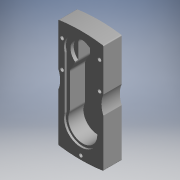
# Autodesk Inventor part: 2610112 EAMM-U-70-D40-...-173---(OT)
Saved by Autodesk Inventor 2017.3 (Build 213256000, 256)
## iProperties
Part Number: 2610112 EAMM-U-70-D40-...-173---(OT)
Material: Generic
Catalog Web Link: www.cadenas.de
Description: EAMM-U---(OT)-Fousing top part
Vendor: FESTO
Document SubType Name: Modeling
Designer: partserver
Manufacturer: FESTO
Mass: 199.697 g
Surface Area: 497.172 cm^2
Volume: 199.697 cm^3
Density: 1 g/cm^3
Appearance: PSOLRGB-192-192-192
Category: PARTsolutions
Company: FESTO
Title: 2610112 EAMM-U-70-D40-...-173---(OT)
Author: Cadenas PARTsolutions
Comments: Fousing top part
PSOL_IDENT_0: {$CADENAS_DATA\23d-libs\festo\parts\e\eamm\parts\eamm_u_ot.prj},220 {VTYP=3D},{NB=2610112 EAMM-U-70-
PSOL_IDENT_1: D40-...-173---(OT)},{LINA=2610112 EAMM-U-70-D40-...-173---(OT)},{NN=EAMM-U---(OT)},{DATE=27.10.2020
PSOL_IDENT_2: 09:44:40},{GEOMDATE=08.01.2020 14:15:00},{VERSION=},{LINEID=520},{WBVAR=},{WBNUMERIC=}  {NB=2610112
PSOL_IDENT_3: EAMM-U-70-D40-...-173---(OT)},{LINA=2610112 EAMM-U-70-D40-...-173---(OT)},{KT=DUMMY},{TNR=2610112},{
PSOL_IDENT_4: TYP=EAMM-U-70-D40-...-173},{VERS=6},{S=0},{B1=38.000},{D=M6},{D1=6.000},{H0=96.000},{H1=38.000},{H5=
PSOL_IDENT_5: 34.500},{H7=0.000},{H8=0.000},{H9=0.000},{H10=0.000},{T1=0.000},{T2=0.000}
NB: 2610112 EAMM-U-70-D40-...-173---(OT)
NN: EAMM-U---(OT)
NT: Fousing top part
NBSYN: $TNR. $TYP.---(OT)
LINA: 2610112 EAMM-U-70-D40-...-173---(OT)
CATALOG: Festo
TNR: 2610112
TYP: EAMM-U-70-D40-...-173
VERS: 6
B1: 38
D: M6
D1: 6
H0: 96
H1: 38
H5: 34.5
H7: 0
H8: 0
H9: 0
H10: 0
T1: 0
T2: 0
SUPPLIER: FESTO
ARTICLENO: 2610112 EAMM-U-70-D40-...-173---(OT)
BOMINFO: 2610112 EAMM-U-70-D40-...-173---(OT)
CREATOR: CADENAS GmbH
Autodesk Inventor part; units mm, degrees
sketch "Sketch_1" plane through (0, 0, 0) normal (0, 1, 0) x (-1, 0, 0)
  line L0 (35, -76.5086) -> (35, -3.969)
  arc A0 (35, -3.969) -> (33.7199, -2.4852) centre (33.5, -3.969) ccw
  arc A1 (33.7199, -2.4852) -> (-33.7199, -2.4852) centre (0, -230) ccw
  arc A2 (-33.7199, -2.4852) -> (-35, -3.969) centre (-33.5, -3.969) ccw
  line L1 (-35, -3.969) -> (-35, -76.5086)
  arc A3 (-35, -76.5086) -> (-34.8767, -77.1042) centre (-33.5, -76.5086) ccw
  arc A4 (-34.8767, -104.8958) -> (-34.8767, -77.1042) centre (-67, -91) ccw
  arc A5 (-34.8767, -104.8958) -> (-35, -105.4914) centre (-33.5, -105.4914) ccw
  line L2 (-35, -105.4914) -> (-35, -169.531)
  arc A6 (-35, -169.531) -> (-33.7199, -171.0148) centre (-33.5, -169.531) ccw
  arc A7 (-33.7199, -171.0148) -> (33.7199, -171.0148) centre (0, 56.5) ccw
  arc A8 (33.7199, -171.0148) -> (35, -169.531) centre (33.5, -169.531) ccw
  line L3 (35, -169.531) -> (35, -105.4914)
  arc A9 (35, -105.4914) -> (34.8767, -104.8958) centre (33.5, -105.4914) ccw
  arc A10 (34.8767, -77.1042) -> (34.8767, -104.8958) centre (67, -91) ccw
  arc A11 (34.8767, -77.1042) -> (35, -76.5086) centre (33.5, -76.5086) ccw
  constraints: 24 point on circle, 12 centre point, 8 end point
extrude "Extrusion1" add sketch "Sketch_1" along normal blind 28.5
sketch "Sketch_2" plane through (0, 0, 0) normal (0, 1, 0) x (-1, 0, 0)
  arc A0 (20.7692, -51.6538) -> (-20.7692, -51.6538) centre (0, -43) ccw
  arc A1 (-20, -55.5) -> (-20.7692, -51.6538) centre (-30, -55.5) ccw
  line L0 (-20, -55.5) -> (-20, -106.3205)
  arc A2 (-20, -106.3205) -> (-18.6603, -111.3205) centre (-10, -106.3205) ccw
  line L1 (-18.6603, -111.3205) -> (-13.3397, -120.5359)
  arc A3 (-12, -125.5359) -> (-13.3397, -120.5359) centre (-22, -125.5359) ccw
  line L2 (-12, -125.5359) -> (-12, -147)
  arc A4 (-12, -147) -> (12, -147) centre (0, -147) ccw
  line L3 (12, -147) -> (12, -125.5359)
  arc A5 (13.3397, -120.5359) -> (12, -125.5359) centre (22, -125.5359) ccw
  line L4 (13.3397, -120.5359) -> (18.6603, -111.3205)
  arc A6 (18.6603, -111.3205) -> (20, -106.3205) centre (10, -106.3205) ccw
  line L5 (20, -106.3205) -> (20, -55.5)
  arc A7 (20.7692, -51.6538) -> (20, -55.5) centre (30, -55.5) ccw
  constraints: 16 point on circle, 12 end point, 8 centre point
extrude "Extrusion2" cut sketch "Sketch_2" along normal blind 26.5
sketch "Sketch_21" plane through (0, 0, 0) normal (0, 1, 0) x (-1, 0, 0)
  arc A0 (7.9881, -156.2392) -> (-7.9881, -156.2392) centre (0, -139) ccw
  arc A1 (-6.6503, -156.9886) -> (-7.9881, -156.2392) centre (-12.1923, -165.3125) ccw
  arc A2 (-6.6503, -156.9886) -> (6.6503, -156.9886) centre (0, -147) ccw
  arc A3 (7.9881, -156.2392) -> (6.6503, -156.9886) centre (12.1923, -165.3125) ccw
  constraints: 8 point on circle, 4 centre point
extrude "Extrusion3" cut sketch "Sketch_21" along normal blind 8
sketch "Sketch_3" plane through (0, 0, 0) normal (0, 1, 0) x (-1, 0, 0)
  arc A0 (25.2778, -49.0856) -> (-25.2778, -49.0856) centre (0, -43) ccw
  arc A1 (-25, -51.4261) -> (-25.2778, -49.0856) centre (-35, -51.4261) ccw
  line L0 (-25, -51.4261) -> (-25, -130.5739)
  arc A2 (-25.2778, -132.9144) -> (-25, -130.5739) centre (-35, -130.5739) ccw
  arc A3 (-25.2778, -132.9144) -> (25.2778, -132.9144) centre (0, -139) ccw
  arc A4 (25, -130.5739) -> (25.2778, -132.9144) centre (35, -130.5739) ccw
  line L1 (25, -130.5739) -> (25, -51.4261)
  arc A5 (25.2778, -49.0856) -> (25, -51.4261) centre (35, -51.4261) ccw
  constraints: 12 point on circle, 6 centre point, 4 end point
extrude "Extrusion4" cut sketch "Sketch_3" along normal blind 3
sketch "Sketch5" plane through (0, 28.5, 0) normal (0, 1, 0) x (1, 0, 0)
  point P0 (0, 6)
hole "Hole1" at (0, 28.5, -6) direction (0, -1, 0) diameter 5.5 depth 28.5 counterbore diameter 10 counterbore depth 6
sketch "Sketch6" plane through (0, 28.5, 0) normal (0, 1, 0) x (1, 0, 0)
  point P0 (29, 106.5)
hole "Hole2" at (29, 28.5, -106.5) direction (0, -1, 0) diameter 5.5 depth 28.5 counterbore diameter 10 counterbore depth 6
sketch "Sketch7" plane through (0, 28.5, 0) normal (0, 1, 0) x (1, 0, 0)
  point P0 (29, 149)
hole "Hole3" at (29, 28.5, -149) direction (0, -1, 0) diameter 5.5 depth 28.5 counterbore diameter 10 counterbore depth 6
sketch "Sketch8" plane through (0, 28.5, 0) normal (0, 1, 0) x (1, 0, 0)
  point P0 (-29, 106.5)
hole "Hole4" at (-29, 28.5, -106.5) direction (0, -1, 0) diameter 5.5 depth 28.5 counterbore diameter 10 counterbore depth 6
sketch "Sketch9" plane through (0, 28.5, 0) normal (0, 1, 0) x (1, 0, 0)
  point P0 (-29, 149)
hole "Hole5" at (-29, 28.5, -149) direction (0, -1, 0) diameter 5.5 depth 28.5 counterbore diameter 10 counterbore depth 6
sketch "Sketch10" plane through (0, 28.5, 0) normal (0, 1, 0) x (1, 0, 0)
  point P0 (19, 158)
hole "Hole6" at (19, 28.5, -158) direction (0, -1, 0) diameter 4.917 depth 16.5 tip angle 120 countersink diameter 6 countersink angle 90 thread size "M6x1" class "6H" standard "ISO Metric profile"
sketch "Sketch11" plane through (0, 28.5, 0) normal (0, 1, 0) x (1, 0, 0)
  point P0 (-19, 158)
hole "Hole7" at (-19, 28.5, -158) direction (0, -1, 0) diameter 4.917 depth 16.5 tip angle 120 countersink diameter 6 countersink angle 90 thread size "M6x1" class "6H" standard "ISO Metric profile"
sketch "Sketch12" plane through (0, 28.5, 0) normal (0, 1, 0) x (1, 0, 0)
  point P0 (19, 120)
hole "Hole8" at (19, 28.5, -120) direction (0, -1, 0) diameter 4.917 depth 16.5 tip angle 120 countersink diameter 6 countersink angle 90 thread size "M6x1" class "6H" standard "ISO Metric profile"
sketch "Sketch13" plane through (0, 28.5, 0) normal (0, 1, 0) x (1, 0, 0)
  point P0 (-19, 120)
hole "Hole9" at (-19, 28.5, -120) direction (0, -1, 0) diameter 4.917 depth 16.5 tip angle 120 countersink diameter 6 countersink angle 90 thread size "M6x1" class "6H" standard "ISO Metric profile"
ref_plane "ANBAU_XY" through (0, 0, -139) normal (0, 1, 0) x (1, 0, 0)
ref_plane "ANBAU_YZ" through (0, 0, -139) normal (1, 0, 0) x (0, 0, -1)
ref_plane "ANBAU_ZX" through (0, 0, -139) normal (0, 0, -1) x (0, 1, 0)
ref_plane "S1_1_XY" through (29, 22.5, -149) normal (0, 1, 0) x (1, 0, 0)
ref_plane "S1_1_YZ" through (29, 22.5, -149) normal (1, 0, 0) x (0, 0, -1)
ref_plane "S1_1_ZX" through (29, 22.5, -149) normal (0, 0, -1) x (0, 1, 0)
ref_plane "S1_2_XY" through (29, 22.5, -106.5) normal (0, 1, 0) x (1, 0, 0)
ref_plane "S1_2_YZ" through (29, 22.5, -106.5) normal (1, 0, 0) x (0, 0, -1)
ref_plane "S1_2_ZX" through (29, 22.5, -106.5) normal (0, 0, -1) x (0, 1, 0)
ref_plane "S2_1_XY" through (-29, 22.5, -149) normal (0, 1, 0) x (1, 0, 0)
ref_plane "S2_1_YZ" through (-29, 22.5, -149) normal (1, 0, 0) x (0, 0, -1)
ref_plane "S2_1_ZX" through (-29, 22.5, -149) normal (0, 0, -1) x (0, 1, 0)
ref_plane "S2_2_XY" through (-29, 22.5, -106.5) normal (0, 1, 0) x (1, 0, 0)
ref_plane "S2_2_YZ" through (-29, 22.5, -106.5) normal (1, 0, 0) x (0, 0, -1)
ref_plane "S2_2_ZX" through (-29, 22.5, -106.5) normal (0, 0, -1) x (0, 1, 0)
ref_plane "S3_XY" through (0, 22.5, -6) normal (0, 1, 0) x (1, 0, 0)
ref_plane "S3_YZ" through (0, 22.5, -6) normal (1, 0, 0) x (0, 0, -1)
ref_plane "S3_ZX" through (0, 22.5, -6) normal (0, 0, -1) x (0, 1, 0)
body "Solid1"
